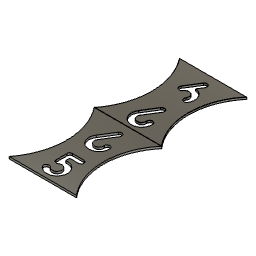
ruler-stencil-5-6 v11 (Autodesk Fusion 360 design; units mm, degrees)
Autodesk Fusion 360 part; units mm, degrees
sketch "Sketch1" plane through (0, 0, 0) normal (0, 0, 1) x (1, 0, 0)
  line L0 (35.966, 13.2447) -> (90.2553, 13.4329) construction
  line L1 (90.2553, 13.4329) -> (90.006, 85.376) construction
  line L2 (90.006, 85.376) -> (35.7166, 85.1879) construction
  line L3 (35.7166, 85.1879) -> (35.966, 13.2447) construction
  arc A0 (83.4029, 53.9289) -> (42.5375, 70.0012) centre (64.1284, 64.9097) ccw
  arc A1 (72.1074, 60.364) -> (83.4029, 53.9289) centre (77.7552, 57.1464) ccw
  arc A2 (72.1074, 60.364) -> (55.1905, 67.0174) centre (64.1284, 64.9097) ccw
  arc A3 (42.5375, 70.0012) -> (55.1905, 67.0174) centre (48.864, 68.5093) ccw
  arc A4 (77.7552, 57.1464) -> (48.864, 68.5093) centre (64.1284, 64.9097) ccw construction
  line L4 (72.8155, 61.3713) -> (40.9019, 24.0589)
  arc A5 (40.9019, 24.0589) -> (50.7812, 15.6091) centre (45.8416, 19.834) ccw
  line L5 (50.7812, 15.6091) -> (82.6948, 52.9215)
  arc A6 (82.6948, 52.9215) -> (72.8155, 61.3713) centre (77.7552, 57.1464) ccw
  line L6 (77.7552, 57.1464) -> (45.8416, 19.834) construction
  line L7 (45.8641, 13.334) -> (81.7759, 13.4585)
  arc A7 (81.7759, 13.4585) -> (81.7309, 26.4584) centre (81.7534, 19.9585) ccw
  line L8 (81.7309, 26.4584) -> (45.819, 26.334)
  arc A8 (45.819, 26.334) -> (45.8641, 13.334) centre (45.8416, 19.834) ccw
  line L9 (45.8416, 19.834) -> (81.7534, 19.9585) construction
  line L10 (35.9242, 113.3399) -> (90, 113.3399) construction
  line L11 (90, 113.3399) -> (90, 185) construction
  line L12 (90, 185) -> (35.9242, 185) construction
  line L13 (35.9242, 185) -> (35.9242, 113.3399) construction
  line L14 (35.908, 213.3415) -> (89.9813, 213.3415) construction
  line L15 (89.9813, 213.3415) -> (89.9813, 284.9983) construction
  line L16 (89.9813, 284.9983) -> (35.908, 284.9983) construction
  line L17 (35.908, 284.9983) -> (35.908, 213.3415) construction
  line L18 (35.9242, 313.3399) -> (90, 313.3399) construction
  line L19 (90, 313.3399) -> (90, 385) construction
  line L20 (90, 385) -> (35.9242, 385) construction
  line L21 (35.9242, 385) -> (35.9242, 313.3399) construction
  line L22 (32.5266, 413.3399) -> (90, 413.3399) construction
  line L23 (90, 413.3399) -> (90, 485) construction
  line L24 (90, 485) -> (32.5266, 485) construction
  line L25 (32.5266, 485) -> (32.5266, 413.3399) construction
  line L26 (133, -100) -> (0, -100)
  line L27 (35.9386, -86.6622) -> (90.0148, -86.6474) construction
  line L28 (90.0148, -86.6474) -> (89.9952, -14.9867) construction
  line L29 (89.9952, -14.9867) -> (35.919, -15.0015) construction
  line L30 (35.919, -15.0015) -> (35.9386, -86.6622) construction
  line L31 (0, -100) -> (133, -100)
  line L32 (133, -100) -> (0, -100)
  line L33 (133, -100) -> (0, -100)
  line L34 (133, -100) -> (0, -100)
  line L35 (64.6043, -22.3346) -> (64.6202, -80.493)
  arc A9 (64.6202, -80.493) -> (77.6202, -80.4895) centre (71.1202, -80.4912) ccw
  line L36 (77.6202, -80.4895) -> (77.6043, -22.331)
  arc A10 (77.6043, -22.331) -> (64.6043, -22.3346) centre (71.1043, -22.3328) ccw
  line L37 (71.1043, -22.3328) -> (71.1202, -80.4912) construction
  line L38 (67.1647, -17.1628) -> (53.122, -27.8637)
  arc A11 (53.122, -27.8637) -> (61.0013, -38.2037) centre (57.0616, -33.0337) ccw
  line L39 (61.0013, -38.2037) -> (75.044, -27.5028)
  arc A12 (75.044, -27.5028) -> (67.1647, -17.1628) centre (71.1043, -22.3328) ccw
  line L40 (71.1043, -22.3328) -> (57.0616, -33.0337) construction
  arc A13 (62.6751, 144.899) -> (43.1442, 175.8213) centre (62.5702, 166.4619) ccw
  arc A14 (62.6119, 157.8989) -> (62.6751, 144.899) centre (62.6435, 151.3989) ccw
  arc A15 (62.6119, 157.8989) -> (54.8558, 170.1787) centre (62.5702, 166.4619) ccw
  arc A16 (43.1442, 175.8213) -> (54.8558, 170.1787) centre (49, 173) ccw
  arc A17 (62.6435, 151.3989) -> (49, 173) centre (62.5702, 166.4619) ccw construction
  arc A18 (40.7814, 125.7599) -> (62.7816, 157.8975) centre (62.2873, 134.6368) ccw
  arc A19 (52.7979, 130.7199) -> (40.7814, 125.7599) centre (46.7897, 128.2399) ccw
  arc A20 (52.7979, 130.7199) -> (62.5054, 144.9004) centre (62.2873, 134.6368) ccw
  arc A21 (62.7816, 157.8975) -> (62.5054, 144.9004) centre (62.6435, 151.3989) ccw
  arc A22 (46.7897, 128.2399) -> (62.6435, 151.3989) centre (62.2873, 134.6368) ccw construction
  line L41 (62.6435, 157.8989) -> (59.3029, 157.8989)
  arc A23 (59.3029, 157.8989) -> (59.3029, 144.8989) centre (59.3029, 151.3989) ccw
  line L42 (59.3029, 144.8989) -> (62.6435, 144.8989)
  arc A24 (62.6435, 144.8989) -> (62.6435, 157.8989) centre (62.6435, 151.3989) ccw
  line L43 (62.6435, 151.3989) -> (59.3029, 151.3989) construction
  line L44 (65.0009, 278.8959) -> (65.0009, 218.8875)
  arc A25 (65.0009, 218.8875) -> (78.0009, 218.8875) centre (71.5009, 218.8875) ccw
  line L45 (78.0009, 218.8875) -> (78.0009, 278.8959)
  arc A26 (78.0009, 278.8959) -> (65.0009, 278.8959) centre (71.5009, 278.8959) ccw
  line L46 (71.5009, 278.8959) -> (71.5009, 218.8875) construction
  line L47 (80.2041, 242.0576) -> (44.9221, 242.0576)
  arc A27 (44.9221, 242.0576) -> (44.9221, 229.0576) centre (44.9221, 235.5576) ccw
  line L48 (44.9221, 229.0576) -> (80.2041, 229.0576)
  arc A28 (80.2041, 229.0576) -> (80.2041, 242.0576) centre (80.2041, 235.5576) ccw
  line L49 (86.7041, 235.5576) -> (38.4221, 235.5576) construction
  line L50 (51.4221, 235.5576) -> (51.4221, 279)
  arc A29 (51.4221, 279) -> (38.4221, 279) centre (44.9221, 279) ccw
  line L51 (38.4221, 279) -> (38.4221, 235.5576)
  arc A30 (38.4221, 235.5576) -> (51.4221, 235.5576) centre (44.9221, 235.5576) ccw
  line L52 (44.9221, 235.5576) -> (44.9221, 279) construction
  line L53 (79, 384.5) -> (52, 384.5)
  arc A31 (52, 384.5) -> (52, 371.5) centre (52, 378) ccw
  line L54 (52, 371.5) -> (79, 371.5)
  arc A32 (79, 371.5) -> (79, 384.5) centre (79, 378) ccw
  line L55 (79, 378) -> (52, 378) construction
  line L56 (45.5, 378) -> (45.5, 352.5192)
  arc A33 (45.5, 352.5192) -> (58.5, 352.5192) centre (52, 352.5192) ccw
  line L57 (58.5, 352.5192) -> (58.5, 378)
  arc A34 (58.5, 378) -> (45.5, 378) centre (52, 378) ccw
  line L58 (52, 378) -> (52, 352.5192) construction
  arc A35 (42.8172, 323.0771) -> (48.2661, 357.8397) centre (62.3086, 337.8303) ccw
  arc A36 (53.1828, 330.9229) -> (42.8172, 323.0771) centre (48, 327) ccw
  arc A37 (53.1828, 330.9229) -> (55.7339, 347.1987) centre (62.3086, 337.8303) ccw
  arc A38 (48.2661, 357.8397) -> (55.7339, 347.1987) centre (52, 352.5192) ccw
  arc A39 (48, 327) -> (52, 352.5192) centre (62.3086, 337.8303) ccw construction
  line L59 (35.9242, 413.3399) -> (90, 413.3399) construction
  line L60 (90, 413.3399) -> (90, 485) construction
  line L61 (90, 485) -> (35.9242, 485) construction
  line L62 (35.9242, 485) -> (35.9242, 413.3399) construction
  line L63 (62.488, 481.445) -> (42.488, 449.445)
  arc A40 (42.488, 449.445) -> (53.512, 442.555) centre (48, 446) ccw
  line L64 (53.512, 442.555) -> (73.512, 474.555)
  arc A41 (73.512, 474.555) -> (62.488, 481.445) centre (68, 478) ccw
  line L65 (68, 478) -> (48, 446) construction
  line L66 (35.9242, 413.3399) -> (90, 413.3399) construction
  line L67 (90, 413.3399) -> (90, 485) construction
  line L68 (90, 485) -> (35.9242, 485) construction
  line L69 (35.9242, 485) -> (35.9242, 413.3399) construction
  line L70 (53.512, 442.555) -> (73.512, 474.555)
  arc A42 (42.488, 449.445) -> (53.512, 442.555) centre (48, 446) ccw
  arc A43 (73.512, 474.555) -> (62.488, 481.445) centre (68, 478) ccw
  line L71 (35.9242, 413.3399) -> (90, 413.3399) construction
  line L72 (90, 413.3399) -> (90, 485) construction
  line L73 (90, 485) -> (35.9242, 485) construction
  line L74 (35.9242, 485) -> (35.9242, 413.3399) construction
  line L75 (68, 478) -> (48, 446) construction
  line L76 (62.488, 481.445) -> (42.488, 449.445)
  arc A44 (53.4404, 442.443) -> (73.5258, 437.4217) centre (62.6117, 436.4468) ccw
  arc A45 (53.4404, 442.443) -> (42.5596, 449.557) centre (48, 446) ccw
  arc A46 (42.5596, 449.557) -> (86.4742, 438.5783) centre (62.6117, 436.4468) ccw
  arc A47 (86.4742, 438.5783) -> (73.5258, 437.4217) centre (80, 438) ccw
  arc A48 (48, 446) -> (80, 438) centre (62.6117, 436.4468) ccw construction
  arc A49 (53.4404, 542.443) -> (42.5596, 549.557) centre (48, 546) ccw
  arc A50 (42.488, 549.445) -> (53.512, 542.555) centre (48, 546) ccw
  line L77 (68, 578) -> (48, 546) construction
  arc A51 (73.512, 574.555) -> (62.488, 581.445) centre (68, 578) ccw
  arc A52 (73.512, 574.555) -> (62.488, 581.445) centre (68, 578) ccw
  line L78 (53.512, 542.555) -> (73.512, 574.555)
  line L79 (62.488, 581.445) -> (42.488, 549.445)
  line L80 (35.9242, 513.3399) -> (90, 513.3399) construction
  line L81 (90, 513.3399) -> (90, 585) construction
  line L82 (90, 585) -> (35.9242, 585) construction
  line L83 (35.9242, 585) -> (35.9242, 513.3399) construction
  line L84 (35.9242, 513.3399) -> (90, 513.3399) construction
  line L85 (90, 513.3399) -> (90, 585) construction
  line L86 (90, 585) -> (35.9242, 585) construction
  line L87 (35.9242, 585) -> (35.9242, 513.3399) construction
  line L88 (35.9242, 513.3399) -> (90, 513.3399) construction
  line L89 (90, 513.3399) -> (90, 585) construction
  line L90 (90, 585) -> (35.9242, 585) construction
  line L91 (35.9242, 585) -> (35.9242, 513.3399) construction
  line L92 (62.488, 581.445) -> (42.488, 549.445)
  arc A53 (42.488, 549.445) -> (53.512, 542.555) centre (48, 546) ccw
  line L93 (68, 578) -> (48, 546) construction
  arc A54 (86.4742, 538.5783) -> (73.5258, 537.4217) centre (80, 538) ccw
  line L94 (53.512, 542.555) -> (73.512, 574.555)
  line L95 (35.9242, 513.3399) -> (90, 513.3399) construction
  line L96 (90, 513.3399) -> (90, 585) construction
  line L97 (90, 585) -> (35.9242, 585) construction
  line L98 (35.9242, 585) -> (35.9242, 513.3399) construction
  arc A55 (42.509, 549.4784) -> (53.491, 542.5216) centre (48, 546) ccw
  line L99 (-19.5194, 304) -> (141.9792, 304)
  line L100 (141.9792, 304) -> (141.9792, 504)
  line L101 (141.9792, 504) -> (-19.5194, 504)
  line L102 (-19.5194, 504) -> (-19.5194, 304) construction
  circle A56 centre (260.371, 404) radius 154.973
  circle A57 centre (-144.6409, 404) radius 162.7146
  line L103 (89.9332, 485.1929) -> (141.9792, 485.1929)
  line L104 (32.5266, 485) -> (-19.5194, 485)
  arc A58 (53.4404, 542.443) -> (42.5596, 549.557) centre (48, 546) ccw
  line L105 (68, 678) -> (48, 646) construction
  line L106 (53.512, 542.555) -> (73.512, 574.555)
  line L107 (53.512, 642.555) -> (73.512, 674.555)
  line L108 (53.512, 542.555) -> (73.512, 574.555)
  arc A59 (73.512, 574.555) -> (62.488, 581.445) centre (68, 578) ccw
  arc A60 (83.1345, 624.0875) -> (42.509, 649.4784) centre (62.7447, 636.6596) ccw
  line L109 (68, 578) -> (48, 546) construction
  arc A61 (42.488, 649.445) -> (53.512, 642.555) centre (48, 646) ccw
  line L110 (35.9242, 613.3399) -> (90, 613.3399) construction
  line L111 (90, 613.3399) -> (90, 685) construction
  line L112 (90, 685) -> (35.9242, 685) construction
  line L113 (35.9242, 685) -> (35.9242, 613.3399) construction
  arc A62 (42.5596, 549.557) -> (86.4742, 538.5783) centre (62.6117, 536.4468) ccw
  arc A63 (53.4404, 542.443) -> (73.5258, 537.4217) centre (62.6117, 536.4468) ccw
  arc A64 (73.512, 674.555) -> (62.488, 681.445) centre (68, 678) ccw
  line L114 (62.488, 581.445) -> (42.488, 549.445)
  line L115 (35.9242, 613.3399) -> (90, 613.3399) construction
  line L116 (90, 613.3399) -> (90, 685) construction
  line L117 (90, 685) -> (35.9242, 685) construction
  line L118 (35.9242, 685) -> (35.9242, 613.3399) construction
  line L119 (35.9242, 613.3399) -> (90, 613.3399) construction
  line L120 (90, 613.3399) -> (90, 685) construction
  line L121 (90, 685) -> (35.9242, 685) construction
  line L122 (35.9242, 685) -> (35.9242, 613.3399) construction
  line L123 (35.9242, 513.3399) -> (90, 513.3399) construction
  line L124 (90, 513.3399) -> (90, 585) construction
  line L125 (90, 585) -> (35.9242, 585) construction
  line L126 (35.9242, 585) -> (35.9242, 513.3399) construction
  line L127 (35.9242, 513.3399) -> (90, 513.3399) construction
  line L128 (90, 513.3399) -> (90, 585) construction
  line L129 (90, 585) -> (35.9242, 585) construction
  line L130 (35.9242, 585) -> (35.9242, 513.3399) construction
  line L131 (62.488, 581.445) -> (42.488, 549.445)
  arc A65 (42.488, 549.445) -> (53.512, 542.555) centre (48, 546) ccw
  arc A66 (72.0689, 630.9104) -> (53.491, 642.5216) centre (62.7447, 636.6596) ccw
  line L132 (68, 678) -> (48, 646) construction
  line L133 (53.512, 642.555) -> (73.512, 674.555)
  arc A67 (48, 546) -> (80, 538) centre (62.6117, 536.4468) ccw construction
  line L134 (62.488, 681.445) -> (42.488, 649.445)
  arc A68 (42.488, 549.445) -> (53.512, 542.555) centre (48, 546) ccw
  arc A69 (53.4404, 642.443) -> (42.5596, 649.557) centre (48, 646) ccw
  arc A70 (77.6017, 627.4989) -> (48, 646) centre (62.7447, 636.6596) ccw construction
  line L135 (68, 578) -> (48, 546) construction
  arc A71 (86.4742, 638.5783) -> (73.5258, 637.4217) centre (80, 638) ccw
  arc A72 (86.4742, 538.5783) -> (73.5258, 537.4217) centre (80, 538) ccw
  arc A73 (73.512, 674.555) -> (62.488, 681.445) centre (68, 678) ccw
  arc A74 (73.512, 574.555) -> (62.488, 581.445) centre (68, 578) ccw
  line L136 (62.488, 681.445) -> (42.488, 649.445)
  line L137 (32.5266, 513.3399) -> (90, 513.3399) construction
  line L138 (90, 513.3399) -> (90, 585) construction
  line L139 (90, 585) -> (32.5266, 585) construction
  line L140 (32.5266, 585) -> (32.5266, 513.3399) construction
  arc A75 (42.488, 649.445) -> (53.512, 642.555) centre (48, 646) ccw
  line L141 (35.9242, 613.3399) -> (90, 613.3399) construction
  line L142 (90, 613.3399) -> (90, 685) construction
  line L143 (90, 685) -> (35.9242, 685) construction
  line L144 (35.9242, 685) -> (35.9242, 613.3399) construction
  line L145 (35.9242, 513.3399) -> (90, 513.3399) construction
  line L146 (90, 513.3399) -> (90, 585) construction
  line L147 (90, 585) -> (35.9242, 585) construction
  line L148 (35.9242, 585) -> (35.9242, 513.3399) construction
  arc A76 (42.509, 649.4784) -> (53.491, 642.5216) centre (48, 646) ccw
  arc A77 (72.0689, 630.9104) -> (83.1345, 624.0875) centre (77.6017, 627.4989) ccw
  circle A78 centre (-144.6409, 604) radius 162.7146
  line L149 (141.9792, 704) -> (-19.5194, 704)
  circle A79 centre (260.371, 604) radius 154.973
  point P0 (35.9242, 213.3399)
  point P1 (90, 213.3399)
  point P2 (35.9242, 285)
  point P3 (90, 285)
  point P4 (35.9242, 213.3399)
  point P5 (90, 213.3399)
  point P6 (35.9242, 285)
  point P7 (90, 285)
  point P8 (35.9242, 313.3399)
  point P9 (35.9242, 313.3399)
  point P10 (90, 313.3399)
  point P11 (90, 385)
  point P12 (35.9242, 385)
  point P13 (90, 313.3399)
  point P14 (35.9242, 385)
  point P15 (90, 385)
  point P16 (35.9242, 413.3399)
  point P17 (35.9242, 485)
  point P18 (90, 485)
  point P19 (35.9242, 413.3399)
  point P20 (90, 485)
  point P21 (35.9242, 485)
  point P22 (35.9242, 413.3399)
  point P23 (90, 413.3399)
  point P24 (35.9242, 485)
  point P25 (90, 413.3399)
  point P26 (90, 413.3399)
  point P27 (90, 485)
  point P28 (35.9242, -86.6601)
  point P29 (35.9242, -15)
  point P30 (90, -15)
  point P31 (35.9242, -15)
  point P32 (35.9242, -86.6601)
  point P33 (90, -15)
  point P34 (35.9242, -15)
  point P35 (35.9242, -86.6601)
  point P36 (90, -86.6601)
  point P37 (90, -15)
  point P38 (35.9242, -15)
  point P39 (90, -86.6601)
  point P40 (35.9242, -86.6601)
  point P41 (90, -86.6601)
  point P42 (90, -86.6601)
  point P43 (90, -15)
  point P44 (35.9242, 413.3399)
  point P45 (35.9242, 485)
  point P46 (35.9242, 413.3399)
  point P47 (90, 413.3399)
  point P48 (35.9242, 485)
  point P49 (90, 413.3399)
  point P50 (90, 413.3399)
  point P51 (90, 485)
  point P52 (35.9242, 413.3399)
  point P53 (89.9332, 485.1929)
  point P54 (35.9242, 485)
  point P55 (90, 485)
  point P56 (90, 485)
  point P57 (35.9242, 413.3399)
  point P58 (90, 485)
  point P59 (35.9242, 485)
  point P60 (89.9332, 485.1929)
  point P61 (35.9242, 413.3399)
  point P62 (90, 413.3399)
  point P63 (35.9242, 485)
  point P64 (90, 413.3399)
  point P65 (90, 413.3399)
  point P66 (35.9242, 485)
  point P67 (35.9242, 413.3399)
  point P68 (35.9242, 413.3399)
  point P69 (35.9242, 485)
  point P70 (35.9242, 413.3399)
  point P71 (90, 413.3399)
  point P72 (35.9242, 485)
  point P73 (90, 413.3399)
  point P74 (90, 413.3399)
  point P75 (90, 485)
  point P76 (35.9242, 413.3399)
  point P77 (90, 485)
  point P78 (35.9242, 485)
  point P79 (90, 485)
  point P80 (90, 585)
  point P81 (35.9242, 513.3399)
  point P82 (90, 585)
  point P83 (35.9242, 585)
  point P84 (90, 585)
  point P85 (90, 513.3399)
  point P86 (90, 513.3399)
  point P87 (35.9242, 585)
  point P88 (35.9242, 513.3399)
  point P89 (35.9242, 513.3399)
  point P90 (35.9242, 585)
  point P91 (90, 513.3399)
  point P92 (90, 513.3399)
  point P93 (35.9242, 585)
  point P94 (35.9242, 513.3399)
  point P95 (90, 585)
  point P96 (35.9242, 513.3399)
  point P97 (90, 585)
  point P98 (35.9242, 585)
  point P99 (90, 585)
  point P100 (35.9242, 513.3399)
  point P101 (35.9242, 585)
  point P102 (90, 513.3399)
  point P103 (90, 513.3399)
  point P104 (90, 585)
  point P105 (35.9242, 513.3399)
  point P106 (90, 585)
  point P107 (35.9242, 585)
  point P108 (90, 585)
  point P109 (35.9242, 513.3399)
  point P110 (90, 513.3399)
  point P111 (35.9242, 585)
  point P112 (90, 513.3399)
  point P113 (90, 513.3399)
  point P114 (35.9242, 585)
  point P115 (35.9242, 513.3399)
  point P116 (35.9242, 513.3399)
  point P117 (35.9242, 585)
  point P118 (35.9242, 513.3399)
  point P119 (90, 513.3399)
  point P120 (35.9242, 585)
  point P121 (90, 513.3399)
  point P122 (90, 513.3399)
  point P123 (90, 585)
  point P124 (35.9242, 513.3399)
  point P125 (90, 585)
  point P126 (35.9242, 585)
  point P127 (90, 585)
  point P128 (35.9242, 685)
  point P129 (89.9332, 585.1929)
  point P130 (90, 613.3399)
  point P131 (35.9242, 513.3399)
  point P132 (90, 613.3399)
  point P133 (90, 613.3399)
  point P134 (35.9242, 685)
  point P135 (35.9242, 685)
  point P136 (35.9242, 613.3399)
  point P137 (35.9242, 685)
  point P138 (90, 613.3399)
  point P139 (35.9242, 613.3399)
  point P140 (35.9242, 685)
  point P141 (35.9242, 613.3399)
  point P142 (35.9242, 613.3399)
  point P143 (90, 613.3399)
  point P144 (32.5266, 585)
  point P145 (90, 685)
  point P146 (35.9242, 613.3399)
  point P147 (90, 685)
  point P148 (89.9332, 585.1929)
  point P149 (35.9242, 585)
  point P150 (90, 513.3399)
  point P151 (90, 513.3399)
  point P152 (35.9242, 513.3399)
  point P153 (35.9242, 513.3399)
  point P154 (90, 513.3399)
  point P155 (35.9242, 585)
  point P156 (35.9242, 513.3399)
  point P157 (35.9242, 585)
  point P158 (35.9242, 585)
  point P159 (90, 613.3399)
  point P160 (90, 685)
  point P161 (90, 585)
  point P162 (35.9242, 513.3399)
  point P163 (90, 513.3399)
  point P164 (35.9242, 585)
  point P165 (90, 513.3399)
  point P166 (90, 513.3399)
  point P167 (90, 613.3399)
  point P168 (90, 513.3399)
  point P169 (35.9242, 585)
  point P170 (90, 513.3399)
  point P171 (90, 513.3399)
  point P172 (90, 585)
  point P173 (35.9242, 513.3399)
  point P174 (89.9332, 585.1929)
  point P175 (35.9242, 585)
  point P176 (90, 585)
  point P177 (90, 685)
  point P178 (35.9242, 613.3399)
  point P179 (90, 685)
  point P180 (90, 585)
  point P181 (35.9242, 513.3399)
  point P182 (90, 585)
  point P183 (35.9242, 685)
  point P184 (90, 685)
  point P185 (90, 685)
  point P186 (35.9242, 613.3399)
  point P187 (90, 685)
  point P188 (35.9242, 685)
  point P189 (90, 685)
  point P190 (90, 613.3399)
  point P191 (90, 613.3399)
  point P192 (35.9242, 685)
  point P193 (35.9242, 613.3399)
  point P194 (35.9242, 613.3399)
  point P195 (35.9242, 685)
  point P196 (90, 613.3399)
  point P197 (90, 613.3399)
  point P198 (35.9242, 685)
  point P199 (35.9242, 613.3399)
  point P200 (90, 685)
  point P201 (35.9242, 685)
  point P202 (90, 685)
  point P203 (35.9242, 613.3399)
  point P204 (35.9242, 685)
  point P205 (90, 613.3399)
  point P206 (35.9242, 513.3399)
  point P207 (35.9242, 585)
  point P208 (35.9242, 513.3399)
  point P209 (90, 513.3399)
  point P210 (35.9242, 585)
  point P211 (90, 513.3399)
  point P212 (90, 513.3399)
  point P213 (90, 585)
  point P214 (35.9242, 513.3399)
  point P215 (90, 685)
  point P216 (35.9242, 613.3399)
  point P217 (90, 585)
  point P218 (90, 585)
  point P219 (35.9242, 585)
  point P220 (35.9242, 513.3399)
  point P221 (35.9242, 585)
  point P222 (90, 585)
  point P223 (35.9242, 513.3399)
  point P224 (90, 585)
  point P225 (35.9242, 585)
  dimension "d3" = 64
  dimension "d4" = 13
  dimension "d5" = 13
  dimension "d6" = 13
  dimension "d9" = 64
  dimension "d10" = 64
  dimension "d14" = 64
  dimension "d19" = 64
  dimension "d22" = 64
  dimension "d23" = 133
  dimension "d25" = 13
  dimension "d26" = 13
  dimension "d29" = 13
  dimension "d30" = 13
  dimension "d31" = 13
  dimension "d32" = 13
  dimension "d33" = 13
  dimension "d35" = 13
  dimension "d36" = 13
  dimension "d37" = 13
  dimension "d38" = 13
  dimension "d39" = 64
  dimension "d42" = 13
  dimension "d43" = 64
  dimension "d44" = 64
  dimension "d49" = 13
  dimension "d50" = 13
  dimension "d51" = 64
  dimension "d52" = 64
  dimension "d53" = 64
  dimension "d54" = 64
  dimension "d59" = 13
  dimension "d64" = 13
  dimension "d65" = 13
  dimension "d66" = 13
  dimension "d70" = 200
  dimension "d71" = 64
  dimension "d72" = 64
  dimension "d73" = 64
  dimension "d74" = 64
  dimension "d75" = 64
  dimension "d76" = 64
  dimension "d77" = 64
  dimension "d78" = 64
  dimension "d79" = 13
  dimension "d80" = 13
  dimension "d81" = 13
  dimension "d82" = 13
  dimension "d83" = 13
  dimension "d84" = 13
  dimension "d85" = 13
  constraint tangent A0 A1
  constraint tangent A1 A2
  constraint tangent A2 A3
  constraint tangent A0 A3
  constraint tangent L4 A5
  constraint tangent A5 L5
  constraint parallel L4 L5
  constraint tangent L5 A6
  constraint tangent L4 A6
  constraint coincident A1.centre A4.start
  constraint tangent L7 A7
  constraint tangent A7 L8
  constraint parallel L7 L8
  constraint tangent L8 A8
  constraint tangent L7 A8
  constraint perpendicular L3 L9
  constraint coincident A5.centre L6.end
  constraint horizontal L33
  constraint horizontal L26
  constraint horizontal L32
  constraint horizontal L34
  constraint horizontal L31
  constraint tangent L35 A9
  constraint tangent A9 L36
  constraint parallel L35 L36
  constraint tangent L36 A10
  constraint tangent L35 A10
  constraint perpendicular L29 L37
  constraint tangent L38 A11
  constraint tangent A11 L39
  constraint parallel L38 L39
  constraint tangent L39 A12
  constraint tangent L38 A12
  constraint coincident A10.centre L37.start
  constraint tangent A13 A14
  constraint tangent A14 A15
  constraint tangent A15 A16
  constraint tangent A13 A16
  constraint tangent A18 A19
  constraint tangent A19 A20
  constraint tangent A20 A21
  constraint tangent A18 A21
  constraint coincident A14.centre A17.start
  constraint tangent L41 A23
  constraint tangent A23 L42
  constraint parallel L41 L42
  constraint tangent L42 A24
  constraint tangent L41 A24
  constraint horizontal L43
  constraint tangent L44 A25
  constraint tangent A25 L45
  constraint parallel L44 L45
  constraint tangent L45 A26
  constraint tangent L44 A26
  constraint tangent L47 A27
  constraint tangent A27 L48
  constraint parallel L47 L48
  constraint tangent L48 A28
  constraint tangent L47 A28
  constraint midpoint A28 L49.start
  constraint midpoint A27 L49.end
  constraint perpendicular L15 L49
  constraint vertical L46
  constraint horizontal L49
  constraint tangent L50 A29
  constraint tangent A29 L51
  constraint parallel L50 L51
  constraint tangent L51 A30
  constraint tangent L50 A30
  constraint perpendicular L16 L52
  constraint coincident A27.centre A30.centre
  constraint tangent L53 A31
  constraint tangent A31 L54
  constraint parallel L53 L54
  constraint tangent L54 A32
  constraint tangent L53 A32
  constraint horizontal L55
  constraint tangent L56 A33
  constraint tangent A33 L57
  constraint parallel L56 L57
  constraint tangent L57 A34
  constraint tangent L56 A34
  constraint perpendicular L55 L58
  constraint coincident A31.centre L55.end
  constraint tangent A35 A36
  constraint tangent A36 A37
  constraint tangent A37 A38
  constraint tangent A35 A38
  constraint coincident A33.centre L58.end
  constraint tangent L63 A40
  constraint tangent A40 L64
  constraint parallel L63 L64
  constraint tangent L64 A41
  constraint tangent L63 A41
  constraint tangent A42 L76
  constraint tangent L70 A42
  constraint parallel L70 L76
  constraint tangent L70 A43
  constraint tangent A43 L76
  constraint tangent A44 A45
  constraint tangent A45 A46
  constraint tangent A46 A47
  constraint tangent A44 A47
  constraint coincident A40.centre L65.end
  constraint tangent A50 L79
  constraint tangent A50 L94
  constraint parallel L79 L94
  constraint tangent A51 L94
  constraint tangent A51 L79
  constraint tangent L92 A53
  constraint tangent L78 A53
  constraint parallel L78 L92
  constraint tangent A52 L78
  constraint tangent A52 L92
  constraint coincident A49.centre A50.centre
  constraint horizontal L99
  constraint vertical L100
  constraint horizontal L101
  constraint vertical L102
  constraint coincident L100.end A56
  constraint coincident L99.end A56
  constraint coincident P60 P53
  constraint coincident L100 L103.end
  constraint perpendicular L100 L103
  constraint coincident L24.end
  constraint coincident L102 L104.end
  constraint perpendicular L102 L104
  constraint equal L103 L104
  constraint tangent L114 A65
  constraint tangent L108 A65
  constraint parallel L108 L114
  constraint tangent L108 A59
  constraint tangent A59 L114
  constraint tangent L131 A68
  constraint tangent L106 A68
  constraint parallel L106 L131
  constraint tangent L106 A74
  constraint tangent L131 A74
  constraint tangent A58 A63
  constraint tangent A58 A62
  constraint tangent A62 A72
  constraint tangent A63 A72
  constraint tangent L134 A75
  constraint tangent L107 A75
  constraint parallel L107 L134
  constraint tangent L107 A64
  constraint tangent A64 L134
  constraint tangent A61 L136
  constraint tangent A61 L133
  constraint parallel L133 L136
  constraint tangent L133 A73
  constraint tangent A73 L136
  constraint coincident L105.end A61.centre
  constraint tangent A60 A77
  constraint tangent A66 A77
  constraint tangent A66 A76
  constraint tangent A60 A76
  constraint coincident P174 P148
  constraint coincident P144
  constraint horizontal L149
  constraint coincident L149.start A79
  measures "d4" diameter of A3
  measures "d5" diameter of A5
  measures "d6" diameter of A7
  measures "d23" distance of L26.end L26.start
  measures "d25" diameter of A9
  measures "d26" diameter of A11
  measures "d29" diameter of A16
  measures "d30" diameter of A21
  measures "d31" diameter of A23
  measures "d32" diameter of A25
  measures "d33" diameter of A27
  measures "d35" diameter of A29
  measures "d36" diameter of A31
  measures "d37" diameter of A33
  measures "d38" diameter of A38
  measures "d42" diameter of A40
  measures "d49" diameter of A42
  measures "d50" diameter of A45
  measures "d59" diameter of A50
  measures "d64" diameter of A53
  measures "d65" diameter of A49
  measures "d66" diameter of A55
  measures "d70" distance of L99.start L101.end
  measures "d79" diameter of A65
  measures "d80" diameter of A68
  measures "d81" diameter of A58
  measures "d82" diameter of A75
  measures "d83" diameter of A61
  measures "d84" diameter of A69
  measures "d85" diameter of A76
extrude "Extrude3" add sketch "Sketch1" along normal blind 5 contours L99 L101 A56 A57 makes body 1
extrude "Extrude5" add sketch "Sketch1" along normal blind 5 contours L101 A78 L149 A79 bodies 1
split "Split1" by curves path "Sketch1" along L99 L100 L101 bodies 1 makes body 2 at (51.3478, 607.9545, 5)
fillet "Fillet1" radius 0.4 1 faces at (51.3478, 607.9545, 5) on bodies 2
fillet "Fillet2" radius 0.4 1 faces at (51.3478, 607.9545, 0) on bodies 2
extrude "Extrude1" [suppressed]
